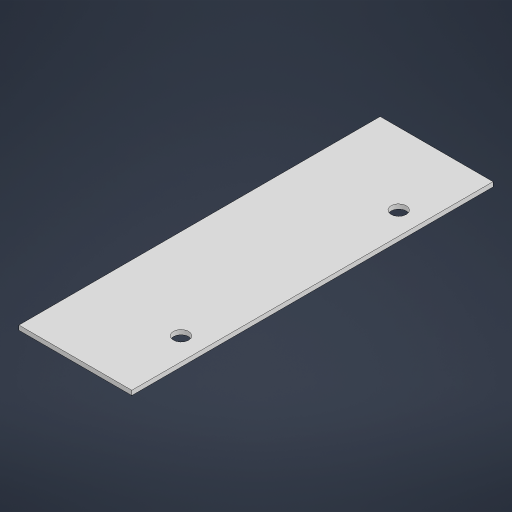
# Autodesk Inventor part: PCB
Saved by Autodesk Inventor 2023 (Build 270158000, 158)
## iProperties
Created: 2024-04-03
Part Number: PCB
Material: Generic
Document SubType Name: Modeling
Designer: Michał
Density: 1 g/cm^3
Appearance: Default
Author: Michał
Autodesk Inventor part; units mm, degrees
ref_plane "YZ Plane" through (0, 0, 0) normal (1, 0, 0) x (0, 1, 0)
ref_plane "XZ Plane" through (0, 0, 0) normal (0, 1, 0) x (-1, 0, 0)
ref_plane "XY Plane" through (0, 0, 0) normal (0, 0, 1) x (1, 0, 0)
sketch "Sketch3" plane through (0, 0, 0) normal (0, 1, 0) x (-1, 0, 0)
  line L0 (0, 0) -> (25, 0)
  line L1 (25, 0) -> (25, -80)
  line L2 (25, -80) -> (0, -80)
  line L3 (0, -80) -> (0, 0)
  dimension "d21" = 25
  dimension "d22" = 80
  constraints: 8 end point, 2 parallel, 1 horizontal, 1 perpendicular
  measures "d21" distance of L0.start L0.end
  measures "d22" distance between parallel lines of L2 L0
extrude "Extrusion2" add sketch "Sketch3" along normal blind 1
sketch "Sketch4" plane through (0, 1, 0) normal (0, 1, 0) x (1, 0, 0)
  line L0 (-25, 80) -> (-25, 0) construction
  line L1 (-25, 40) -> (0, 40) construction
  line L2 (0, 0) -> (0, 80) construction
  point P0 (-5, 15.9)
  point P1 (-5, 64.1)
  dimension "d25" = 5
  dimension "d26" = 48.2
  constraints: 2 end point, 2 midpoint, 1 symmetric about line, 1 vertical alignment
  measures "d25" distance from line of L2 point (-5, 64.1)
  measures "d26" distance of point (-5, 15.9) point (-5, 64.1)
hole "Hole2" at (-5, 1, -15.9) at (-5, 1, -64.1) direction (0, -1, 0) diameter 3.4 end through all clearance for "Countersunk Flat Head Screw ISO 2009/7046" size "M3" standard "ISO"
body "Solid2"
